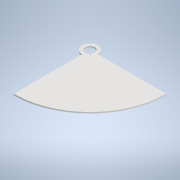
# Autodesk Inventor part: ramp
Saved by Autodesk Inventor 2021 (Build 250183000, 183)
## iProperties
Created: 2020-09-12
Part Number: ramp
Material: Generic
Document SubType Name: Modeling
Designer: deli
Density: 1 g/cm^3
Appearance: Default
Author: deli
Autodesk Inventor part; units mm, degrees
ref_plane "YZ Plane" through (0, 0, 0) normal (1, 0, 0) x (0, 1, 0)
ref_plane "XZ Plane" through (0, 0, 0) normal (0, 1, 0) x (-1, 0, 0)
ref_plane "XY Plane" through (0, 0, 0) normal (0, 0, 1) x (1, 0, 0)
sketch "Sketch1" plane through (0, 0, 0) normal (0, 1, 0) x (-1, 0, 0)
  arc A0 (40.8631, 289.0847) -> (-143.2869, 104.9347) centre (40.8631, 104.9347) ccw
  line L0 (21.8131, 104.9347) -> (-143.2869, 104.9347)
  line L1 (40.8631, 289.0847) -> (40.8631, 123.9847)
  arc A1 (21.8131, 104.9347) -> (40.8631, 123.9847) centre (40.8631, 104.9347) ccw
  point P0 (0, 0)
  dimension "d0" = 368.3
  dimension "d2" = 0
  dimension "d3" = 38.1
  constraints: 4 end point, 4 point on circle, 2 centre point, 1 horizontal, 1 vertical
  measures "d0" diameter of A0
  measures "d2" distance from line of A0.centre L0
  measures "d3" diameter of A1
extrude "Extrusion1" add sketch "Sketch1" along normal blind 3.175
sketch "Sketch2" plane through (0, 3.175, 0) normal (0, 1, 0) x (1, 0, 0)
  circle A0 centre (-30.9636, -95.0352) radius 1.25 projected
  circle A1 centre (-30.9636, -114.8342) radius 1.25 projected
  circle A2 centre (-50.7626, -114.8342) radius 1.25 projected
  circle A3 centre (-50.7626, -95.0352) radius 1.25 projected
  circle A4 centre (-50.7626, -114.8342) radius 0.996
  circle A5 centre (-30.9636, -114.8342) radius 0.996
  circle A6 centre (-30.9636, -95.0352) radius 0.996
  circle A7 centre (-50.7626, -95.0352) radius 0.996
  arc A8 (-21.8131, -104.9347) -> (-40.8631, -123.9847) centre (-40.8631, -104.9347) ccw projected
  circle A9 centre (-40.8631, -104.9347) radius 11.43
  point P0 (0, 0)
  dimension "d6" = 2.5
  dimension "d7" = 1.992
  dimension "d8" = 1.992
  dimension "d9" = 1.992
  dimension "d10" = 1.992
  dimension "d11" = 22.86
  constraints: 5 centre point, 5 coincident
  measures "d6" diameter of A2
  measures "d7" diameter of A4
  measures "d8" diameter of A7
  measures "d9" diameter of A6
  measures "d10" diameter of A5
  measures "d11" diameter of A9
extrude "Extrusion2" cut sketch "Sketch2" against normal blind 3.175 contours A4 | A5 | A6 | A7 | A9
sketch "Sketch3" plane through (0, 3.175, 0) normal (0, 1, 0) x (1, 0, 0)
  arc A0 (-40.8631, -289.0847) -> (143.2869, -104.9347) centre (-40.8631, -104.9347) ccw projected
  circle A1 centre (-40.8631, -104.9347) radius 185.7375
  line L0 (143.2869, -104.9347) -> (144.8744, -104.9347)
  line L1 (-40.8631, -123.9847) -> (-40.8631, -289.0847) projected
  line L2 (-40.8631, -289.0847) -> (-40.8631, -290.6722)
  point P0 (0, 0)
  dimension "d14" = 184.15
  dimension "d15" = 371.475
  constraints: 4 end point, 2 point on circle, 1 centre point, 1 coincident, 1 horizontal, 1 vertical
  measures "d14" radius of A0
  measures "d15" diameter of A1
extrude "Extrusion3" add sketch "Sketch3" along normal blind 25.4 and the other way blind 3.175 contours A0 L0 A1 L2 picked at (143.7515, -117.0198)
body "Solid1"
